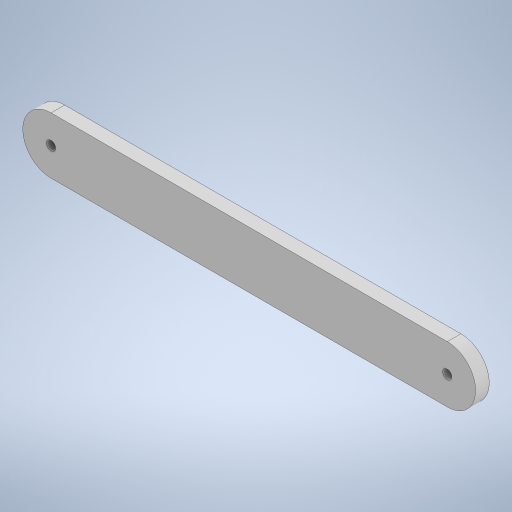
# Autodesk Inventor part: Horizontal
Saved by Autodesk Inventor 2024 (Build 280153000, 153)
## iProperties
Created: 2024-03-09
Part Number: Horizontal
Material: Generic
Document SubType Name: Modeling
Designer: ddcos
Density: 1 g/cm^3
Appearance: Default
Author: ddcos
Autodesk Inventor part; units mm, degrees
ref_plane "YZ Plane" through (0, 0, 0) normal (1, 0, 0) x (0, 1, 0)
ref_plane "XZ Plane" through (0, 0, 0) normal (0, 1, 0) x (-1, 0, 0)
ref_plane "XY Plane" through (0, 0, 0) normal (0, 0, 1) x (1, 0, 0)
sketch "Sketch1" plane through (0, 0, 0) normal (0, 0, 1) x (1, 0, 0)
  line L0 (0, 0) -> (-250, 0)
  line L1 (-250, 0) -> (-250, 25)
  line L2 (-250, 25) -> (0, 25)
  line L3 (0, 25) -> (0, 0)
  dimension "d0" = 250
  dimension "d1" = 25
  constraints: 8 end point, 2 parallel, 1 horizontal, 1 perpendicular
  measures "d0" distance of L1.end L2.end
  measures "d1" distance of L2.end L0.start
extrude "Extrusion1" add sketch "Sketch1" along normal blind 25
sketch "Sketch3" plane through (0, 0, 25) normal (0, 0, 1) x (1, 0, 0)
  line L0 (0, 25) -> (-250, 25) projected
  line L1 (-250, 0) -> (0, 0) projected
  line L2 (-250, 25) -> (-200, 25)
  line L3 (-200, 25) -> (-200, 0)
  line L4 (-200, 0) -> (-250, 0)
  line L5 (-250, 0) -> (-250, 25)
  dimension "d13" = 50
  constraints: 8 end point, 2 parallel, 1 horizontal, 1 perpendicular, 1 point on line
  measures "d13" distance of L3.end L4.end
extrude "Extrusion3" cut sketch "Sketch3" against normal blind 25
sketch "Sketch4" plane through (0, 0, 25) normal (0, 0, 1) x (1, 0, 0)
  circle A0 centre (-187.5, 12.5) radius 12.5
  line L0 (-200, 0) -> (0, 0) projected
  line L1 (-200, 25) -> (-200, 0) projected
  circle A1 centre (-187.5, 12.5) radius 2
  circle A2 centre (-12.5, 12.5) radius 12.5
  line L2 (0, 0) -> (0, 25) projected
  circle A3 centre (-12.5, 12.5) radius 2
  line L3 (0, 25) -> (-200, 25) projected
  point P0 (-12.5, 25)
  point P1 (0, 12.5)
  point P2 (-12.5, 0)
  point P3 (-187.5, 25)
  point P4 (-200, 12.5)
  point P5 (-187.5, 0)
  dimension "d16" = 25
  dimension "d17" = 12.5
  dimension "d18" = 12.5
  dimension "d19" = 4
  dimension "d20" = 25
  dimension "d21" = 12.5
  dimension "d22" = 12.5
  dimension "d23" = 4
  constraints: 4 centre point, 2 coincident
  measures "d16" diameter of A0
  measures "d17" distance from line of L0 A0.centre
  measures "d18" distance from line of L1 A0.centre
  measures "d19" diameter of A1
  measures "d20" diameter of A2
  measures "d21" distance from line of L2 A2.centre
  measures "d22" distance from line of L0 A2.centre
  measures "d23" diameter of A3
extrude "Extrusion4" cut sketch "Sketch4" against normal blind 25 contours A0 L1 L3 | L0 L1 A0 | L3 L2 A2 | A2 L2 L0 | A1 | A3
sketch "Sketch5" plane through (-187.5, 25, 0) normal (0, 1, 0) x (1, 0, 0)
  line L0 (-12.5, 0) -> (-12.5, -25) projected
  line L1 (187.5, 0) -> (-12.5, 0)
  line L2 (-12.5, 0) -> (-12.5, -19)
  line L3 (-12.5, -19) -> (187.5, -19)
  line L4 (187.5, -19) -> (187.5, 0)
  dimension "d26" = 19
  constraints: 8 end point, 2 parallel, 1 horizontal, 1 perpendicular, 1 point on line
  measures "d26" distance between parallel lines of L1 L3
extrude "Extrusion5" cut sketch "Sketch5" against normal blind 100
body "Solid1"
